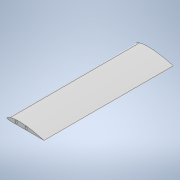
# Autodesk Inventor part: полукрыло
Saved by Autodesk Inventor 2022.1 (Build 261234000, 234)
## iProperties
Created: 2021-12-25
Part Number: полукрыло
Material: Типовые
Document SubType Name: Modeling
Designer: Grigori
Density: 1 g/cm^3
Appearance: По умолчанию
Author: Grigori
Autodesk Inventor part; units mm, degrees
ref_plane "YZ Plane" through (0, 0, 0) normal (1, 0, 0) x (0, 1, 0)
ref_plane "XZ Plane" through (0, 0, 0) normal (0, 1, 0) x (-1, 0, 0)
ref_plane "XY Plane" through (0, 0, 0) normal (0, 0, 1) x (1, 0, 0)
sketch "Эскиз1" plane through (0, 0, 0) normal (0, 0, 1) x (1, 0, 0)
  spline S0 degree 3 poles (150, 0) (149.8103, 0.0535) (149.6206, 0.107) (149.4309, 0.1604) (148.6924, 0.3681) (147.9536, 0.5746) (147.2145, 0.7798) (146.4753, 0.985) (145.7358, 1.1888) (144.996, 1.3912) (143.8986, 1.6914) (142.8004, 1.9884) (141.7013, 2.2822) (141.3183, 2.3846) (140.9352, 2.4865) (140.552, 2.5881) (139.0691, 2.9811) (137.5846, 3.368) (136.0985, 3.7487) (135.1897, 3.9814) (134.2803, 4.2119) (133.3703, 4.4399) (132.7921, 4.5848) (132.2137, 4.7287) (131.635, 4.8717) (128.6558, 5.6077) (125.6697, 6.318) (122.6779, 7.0005) (120.6568, 7.4616) (118.6331, 7.91) (116.6066, 8.3452) (115.6332, 8.5543) (114.6592, 8.7603) (113.6845, 8.9631) (111.8511, 9.3447) (110.0153, 9.7153) (108.1768, 10.0742) (107.0035, 10.3033) (105.8291, 10.5276) (104.6538, 10.7471) (103.0086, 11.0542) (101.3616, 11.3518) (99.7134, 11.639) (98.3391, 11.8786) (96.9638, 12.111) (95.5877, 12.336) (92.5615, 12.8308) (89.5317, 13.2894) (86.4974, 13.7081) (85.2382, 13.8819) (83.9782, 14.0488) (82.7174, 14.2084) (80.9402, 14.4335) (79.1615, 14.6442) (77.3811, 14.8395) (76.3163, 14.9564) (75.2508, 15.0677) (74.1847, 15.1733) (72.2039, 15.3694) (70.2207, 15.5457) (68.2355, 15.7002) (67.3658, 15.7679) (66.4958, 15.8315) (65.6252, 15.8907) (63.4387, 16.0393) (61.2497, 16.1605) (59.0563, 16.2511) (58.383, 16.2789) (57.7092, 16.3039) (57.0352, 16.3258) (56.1747, 16.3538) (55.3136, 16.3769) (54.4524, 16.3949) (53.8776, 16.4069) (53.3029, 16.4166) (52.7283, 16.4239) (51.7678, 16.4362) (50.8078, 16.4419) (49.8487, 16.4407) (49.3747, 16.4401) (48.901, 16.4378) (48.4274, 16.4338) (45.8405, 16.4119) (43.2596, 16.3383) (40.6856, 16.2053) (40.41, 16.191) (40.1345, 16.1761) (39.859, 16.1605) (38.6139, 16.0899) (37.3704, 16.0052) (36.1287, 15.9051) (34.6132, 15.783) (33.1004, 15.6381) (31.5904, 15.468) (31.5076, 15.4587) (31.4248, 15.4493) (31.342, 15.4398) (29.9162, 15.2766) (28.4929, 15.0908) (27.0726, 14.8799) (25.6743, 14.6724) (24.2789, 14.4406) (22.8866, 14.1816) (22.7835, 14.1625) (22.6805, 14.1432) (22.5775, 14.1237) (21.8305, 13.9826) (21.0845, 13.8337) (20.3393, 13.6764) (19.5946, 13.5192) (18.8507, 13.3537) (18.1079, 13.1792) (17.3655, 13.0048) (16.6241, 12.8214) (15.8838, 12.6285) (15.5138, 12.5321) (15.144, 12.4333) (14.7746, 12.3319) (14.6856, 12.3074) (14.5965, 12.2828) (14.5075, 12.2582) knots 0 0 0 0 0.004293 0.004293 0.004293 0.021004 0.021004 0.021004 0.037715 0.037715 0.037715 0.0625 0.0625 0.0625 0.071137 0.071137 0.071137 0.104561 0.104561 0.104561 0.125 0.125 0.125 0.137985 0.137985 0.137985 0.204838 0.204838 0.204838 0.25 0.25 0.25 0.271693 0.271693 0.271693 0.3125 0.3125 0.3125 0.338544 0.338544 0.338544 0.375 0.375 0.375 0.4054 0.4054 0.4054 0.472254 0.472254 0.472254 0.5 0.5 0.5 0.539109 0.539109 0.539109 0.5625 0.5625 0.5625 0.605962 0.605962 0.605962 0.625 0.625 0.625 0.672821 0.672821 0.672821 0.6875 0.6875 0.6875 0.706241 0.706241 0.706241 0.71875 0.71875 0.71875 0.739664 0.739664 0.739664 0.75 0.75 0.75 0.806455 0.806455 0.806455 0.8125 0.8125 0.8125 0.839823 0.839823 0.839823 0.873171 0.873171 0.873171 0.875 0.875 0.875 0.906495 0.906495 0.906495 0.9375 0.9375 0.9375 0.939794 0.939794 0.939794 0.956434 0.956434 0.956434 0.973065 0.973065 0.973065 0.989689 0.989689 0.989689 0.997997 0.997997 0.997997 1 1 1 1
  spline S1 degree 3 poles (14.5075, 12.2582) (14.4875, 12.2539) (14.4676, 12.2496) (14.4477, 12.2453) (14.427, 12.2408) (14.4064, 12.2362) (14.3858, 12.2315) (14.3651, 12.2269) (14.3445, 12.2221) (14.324, 12.2172) (14.3132, 12.2146) (14.3023, 12.212) (14.2915, 12.2094) (14.2612, 12.202) (14.231, 12.1944) (14.2008, 12.1867) (14.1599, 12.1761) (14.119, 12.1653) (14.0782, 12.1541) (14.0577, 12.1485) (14.0372, 12.1429) (14.0168, 12.1371) (13.9965, 12.1315) (13.9762, 12.1257) (13.9559, 12.1199) (13.8954, 12.1024) (13.835, 12.0844) (13.7749, 12.066) (13.7541, 12.0596) (13.7333, 12.0531) (13.7125, 12.0467) (13.653, 12.0281) (13.5937, 12.0092) (13.5344, 11.99) (13.4322, 11.9569) (13.3302, 11.923) (13.2285, 11.8884) (13.0674, 11.8337) (12.9069, 11.7774) (12.7469, 11.7195) (12.6917, 11.6995) (12.6365, 11.6794) (12.5813, 11.659) (12.4766, 11.6204) (12.372, 11.5811) (12.2677, 11.5412) (12.1086, 11.4804) (11.95, 11.4184) (11.792, 11.3554) (11.7416, 11.3353) (11.6912, 11.3151) (11.6409, 11.2948) (11.3758, 11.1877) (11.1122, 11.078) (10.8499, 10.966) (10.8042, 10.9465) (10.7585, 10.9269) (10.7129, 10.9072) (10.4469, 10.7925) (10.1823, 10.6754) (9.9188, 10.5559) (9.6102, 10.416) (9.3033, 10.2729) (8.9981, 10.1267) (8.9613, 10.1091) (8.9246, 10.0914) (8.8879, 10.0738) (8.6197, 9.9445) (8.3528, 9.8129) (8.0873, 9.6788) (7.7854, 9.5263) (7.4851, 9.3707) (7.1867, 9.2117) (7.1586, 9.1967) (7.1305, 9.1817) (7.1024, 9.1666) (6.8324, 9.022) (6.5639, 8.8747) (6.2971, 8.7242) (6.0025, 8.5581) (5.7099, 8.3882) (5.4196, 8.214) (5.3998, 8.2021) (5.38, 8.1902) (5.3603, 8.1783) (5.09, 8.0155) (4.8218, 7.8489) (4.556, 7.6779) (4.5403, 7.6678) (4.5246, 7.6576) (4.5088, 7.6475) (4.2396, 7.4736) (3.9729, 7.2951) (3.709, 7.1108) (3.6972, 7.1026) (3.6855, 7.0944) (3.6737, 7.0861) (3.4065, 6.8987) (3.1421, 6.7053) (2.8827, 6.5047) (2.8749, 6.4987) (2.867, 6.4926) (2.8591, 6.4865) (2.7317, 6.3876) (2.6054, 6.2869) (2.4809, 6.1845) (2.3488, 6.0758) (2.2188, 5.9652) (2.091, 5.8521) (2.0869, 5.8485) (2.0828, 5.8449) (2.0788, 5.8413) (1.9528, 5.7295) (1.8291, 5.6155) (1.7083, 5.4986) (1.5874, 5.3817) (1.4693, 5.2619) (1.3549, 5.1385) (1.2404, 5.0151) (1.1297, 4.8881) (1.0237, 4.7556) (0.9692, 4.6876) (0.9161, 4.6183) (0.8647, 4.5475) (0.8159, 4.4804) (0.7687, 4.412) (0.7238, 4.3425) (0.7219, 4.3396) (0.72, 4.3367) (0.7182, 4.3338) (0.6716, 4.2613) (0.6274, 4.1875) (0.5864, 4.1119) (0.5482, 4.0415) (0.5127, 3.9696) (0.4805, 3.8956) (0.4782, 3.8903) (0.4759, 3.8851) (0.4737, 3.8798) (0.4424, 3.8065) (0.4146, 3.7313) (0.3921, 3.6549) (0.3901, 3.6483) (0.3882, 3.6416) (0.3864, 3.635) (0.3651, 3.5595) (0.3494, 3.4827) (0.3417, 3.4046) (0.3409, 3.3966) (0.3402, 3.3886) (0.3395, 3.3806) (0.3362, 3.3373) (0.3354, 3.2934) (0.3377, 3.2501) (0.3388, 3.2285) (0.3407, 3.207) (0.3434, 3.1856) (0.345, 3.1732) (0.3469, 3.1609) (0.349, 3.1486) (0.3505, 3.1397) (0.3522, 3.1307) (0.354, 3.1218) (0.3583, 3.1006) (0.3634, 3.0795) (0.3693, 3.0586) (0.3726, 3.047) (0.3761, 3.0355) (0.3799, 3.024) (0.3829, 3.0147) (0.3861, 3.0055) (0.3894, 2.9964) (0.3934, 2.9854) (0.3977, 2.9746) (0.4021, 2.9638) (0.4059, 2.9546) (0.4099, 2.9454) (0.414, 2.9363) (0.4187, 2.926) (0.4235, 2.9157) (0.4285, 2.9056) (0.433, 2.8965) (0.4376, 2.8874) (0.4424, 2.8784) (0.4475, 2.8687) (0.4528, 2.859) (0.4582, 2.8495) (0.4739, 2.8219) (0.4907, 2.7951) (0.5086, 2.7689) (0.5264, 2.7427) (0.5452, 2.7172) (0.5648, 2.6921) (0.5718, 2.6831) (0.5789, 2.6742) (0.5861, 2.6654) (0.6058, 2.6413) (0.6262, 2.6176) (0.6473, 2.5945) (0.6554, 2.5856) (0.6636, 2.5767) (0.6719, 2.568) (0.693, 2.5457) (0.7146, 2.5239) (0.7367, 2.5026) (0.7456, 2.4939) (0.7547, 2.4853) (0.7638, 2.4768) (0.8171, 2.427) (0.8726, 2.3799) (0.9298, 2.335) (0.9405, 2.3266) (0.9513, 2.3182) (0.9621, 2.31) (1.019, 2.2666) (1.0774, 2.2253) (1.1366, 2.1855) (1.1488, 2.1774) (1.1611, 2.1692) (1.1733, 2.1612) (1.3029, 2.0763) (1.4366, 1.9991) (1.5734, 1.9271) (1.5883, 1.9193) (1.6033, 1.9115) (1.6184, 1.9038) (1.7539, 1.834) (1.8924, 1.7693) (2.0326, 1.7086) (2.0503, 1.7009) (2.0679, 1.6933) (2.0856, 1.6858) (2.2242, 1.6269) (2.3643, 1.5718) (2.5053, 1.5198) (2.5253, 1.5124) (2.5454, 1.5051) (2.5655, 1.4978) (2.7268, 1.4394) (2.8893, 1.385) (3.0527, 1.3337) (3.1915, 1.2901) (3.331, 1.2488) (3.4711, 1.2094) (3.496, 1.2024) (3.5208, 1.1955) (3.5457, 1.1886) (3.847, 1.1054) (4.1511, 1.0307) (4.4564, 0.9625) (4.4861, 0.9558) (4.5157, 0.9493) (4.5454, 0.9428) (4.8466, 0.8768) (5.1489, 0.817) (5.4516, 0.762) (5.4857, 0.7558) (5.5199, 0.7497) (5.5541, 0.7436) (5.8524, 0.6906) (6.1511, 0.6422) (6.4502, 0.5976) (6.4888, 0.5918) (6.5275, 0.5861) (6.5662, 0.5805) (6.8609, 0.5374) (7.156, 0.498) (7.4515, 0.4615) (7.4946, 0.4562) (7.5378, 0.4509) (7.581, 0.4457) (7.8721, 0.4107) (8.1634, 0.3785) (8.455, 0.3487) (8.5026, 0.3438) (8.5503, 0.339) (8.598, 0.3343) (9.2202, 0.2724) (9.8433, 0.2213) (10.4673, 0.1785) (10.524, 0.1746) (10.5807, 0.1708) (10.6374, 0.167) (11.2526, 0.1262) (11.8686, 0.0933) (12.4852, 0.0665) (12.5509, 0.0637) (12.6166, 0.0609) (12.6823, 0.0582) (13.0236, 0.0441) (13.3649, 0.0317) (13.7065, 0.0212) (13.9734, 0.0131) (14.2404, 0.0062) (14.5075, 0) knots 0 0 0 0 0.001887 0.001887 0.001887 0.003846 0.003846 0.003846 0.005805 0.005805 0.005805 0.006836 0.006836 0.006836 0.009726 0.009726 0.009726 0.013653 0.013653 0.013653 0.015625 0.015625 0.015625 0.017585 0.017585 0.017585 0.023437 0.023437 0.023437 0.02546 0.02546 0.02546 0.03125 0.03125 0.03125 0.041235 0.041235 0.041235 0.05704 0.05704 0.05704 0.0625 0.0625 0.0625 0.072872 0.072872 0.072872 0.088701 0.088701 0.088701 0.09375 0.09375 0.09375 0.120362 0.120362 0.120362 0.125 0.125 0.125 0.152027 0.152027 0.152027 0.183689 0.183689 0.183689 0.1875 0.1875 0.1875 0.215352 0.215352 0.215352 0.247015 0.247015 0.247015 0.25 0.25 0.25 0.278679 0.278679 0.278679 0.310342 0.310342 0.310342 0.3125 0.3125 0.3125 0.342004 0.342004 0.342004 0.34375 0.34375 0.34375 0.373668 0.373668 0.373668 0.375 0.375 0.375 0.405329 0.405329 0.405329 0.40625 0.40625 0.40625 0.421167 0.421167 0.421167 0.436994 0.436994 0.436994 0.4375 0.4375 0.4375 0.453125 0.453125 0.453125 0.46875 0.46875 0.46875 0.484375 0.484375 0.484375 0.492398 0.492398 0.492398 0.5 0.5 0.5 0.50032 0.50032 0.50032 0.508241 0.508241 0.508241 0.515625 0.515625 0.515625 0.51615 0.51615 0.51615 0.523438 0.523438 0.523438 0.524067 0.524067 0.524067 0.53125 0.53125 0.53125 0.531985 0.531985 0.531985 0.53595 0.53595 0.53595 0.537925 0.537925 0.537925 0.539062 0.539062 0.539062 0.539895 0.539895 0.539895 0.54187 0.54187 0.54187 0.542969 0.542969 0.542969 0.543859 0.543859 0.543859 0.544922 0.544922 0.544922 0.545839 0.545839 0.545839 0.546875 0.546875 0.546875 0.547813 0.547813 0.547813 0.548828 0.548828 0.548828 0.551758 0.551758 0.551758 0.554688 0.554688 0.554688 0.555733 0.555733 0.555733 0.558594 0.558594 0.558594 0.559697 0.559697 0.559697 0.5625 0.5625 0.5625 0.563643 0.563643 0.563643 0.570312 0.570312 0.570312 0.57156 0.57156 0.57156 0.578125 0.578125 0.578125 0.579477 0.579477 0.579477 0.59375 0.59375 0.59375 0.595309 0.595309 0.595309 0.609375 0.609375 0.609375 0.611144 0.611144 0.611144 0.625 0.625 0.625 0.626971 0.626971 0.626971 0.642803 0.642803 0.642803 0.65625 0.65625 0.65625 0.658635 0.658635 0.658635 0.6875 0.6875 0.6875 0.690302 0.690302 0.690302 0.71875 0.71875 0.71875 0.721961 0.721961 0.721961 0.75 0.75 0.75 0.753625 0.753625 0.753625 0.78125 0.78125 0.78125 0.785287 0.785287 0.785287 0.8125 0.8125 0.8125 0.816949 0.816949 0.816949 0.875 0.875 0.875 0.880274 0.880274 0.880274 0.9375 0.9375 0.9375 0.943598 0.943598 0.943598 0.97526 0.97526 0.97526 1 1 1 1
  arc A0 (14.5075, 0) -> (17.2168, 0) centre (15.8621, 58.4021) ccw
  line L0 (150, 0) -> (17.2168, 0)
  line L1 (16.1571, 0) -> (24.1571, 0)
  point P0 (0, 0)
  constraints: 4 end point, 2 point on circle, 1 centre point, 1 point on line, 6 other
extrude "Выдавливание1" add sketch "Эскиз1" along normal blind 520
sketch "Эскиз2" plane through (0, 0, 0) normal (0, 0, -1) x (-1, 0, 0)
  point P0 (0, 0)
sketch "Эскиз3" plane through (0, 0, 520) normal (0, 0, 1) x (1, 0, 0)
  line L0 (56.9547, 0) -> (61.9547, 0) construction
  circle A0 centre (38.5008, 8) radius 5
  circle A1 centre (78.7009, 8) radius 5
  dimension "d4" = 10
  constraints: 2 centre point, 2 end point, 1 horizontal
  measures "d4" diameter of A1
extrude "Выдавливание2" cut sketch "Эскиз3" against normal blind 200
